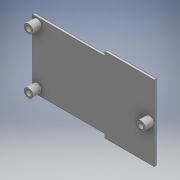
# Autodesk Inventor part: TopChassis
Saved by Autodesk Inventor 2016 (Build 200138000, 138)
## iProperties
Created: 2016-02-18
Part Number: TopChassis
Material: Generic
Document SubType Name: Modeling
Designer: mkepler
Density: 1 g/cm^3
Appearance: Default
Author: mkepler
Autodesk Inventor part; units mm, degrees
ref_plane "YZ Plane" through (0, 0, 0) normal (1, 0, 0) x (0, 1, 0)
ref_plane "XZ Plane" through (0, 0, 0) normal (0, 1, 0) x (-1, 0, 0)
ref_plane "XY Plane" through (0, 0, 0) normal (0, 0, 1) x (1, 0, 0)
sketch "Sketch1" plane through (0, 0, 0) normal (0, 1, 0) x (-1, 0, 0)
  line L0 (0, 0) -> (56, 0)
  line L1 (137.742, -4.5) -> (137.742, -80.5)
  line L2 (56, -85) -> (0, -85)
  line L3 (0, -85) -> (0, 0)
  line L4 (0, 0) -> (56, 0)
  line L5 (56, 0) -> (56, -4.5)
  line L6 (56, -85) -> (56, -80.5)
  line L7 (56, -80.5) -> (137.742, -80.5)
  line L8 (56, -4.5) -> (137.742, -4.5)
  line L9 (56, 0) -> (56, -4.5)
  line L10 (56, -80.5) -> (56, -85)
  dimension "d19" = 56
  dimension "d20" = 4.5
  dimension "d21" = 4.5
  dimension "d54" = 76
  dimension "d55" = 81.742
  dimension "d56" = 85
  constraints: 22 end point, 6 perpendicular, 1 horizontal, 1 vertical
  measures "d19" distance of L0.end L0.start
  measures "d20" distance of L0.end L5.end
  measures "d21" distance of L2.start L6.end
  measures "d54" distance between parallel lines of L7 L8
  measures "d55" distance between parallel lines of L1 L6
  measures "d56" distance between parallel lines of L2 L0
extrude "Extrusion1" add sketch "Sketch1" along normal blind 2.5
sketch "Sketch3" plane through (0, 2.5, 0) normal (0, 1, 0) x (1, 0, 0)
  line L0 (-56, 85) -> (-56, 80.5) projected
  line L1 (0, 0) -> (0, 85) projected
  circle A0 centre (-131.742, 10.5) radius 2.2
  line L2 (-137.742, 80.5) -> (-137.742, 4.5) projected
  line L3 (-137.742, 4.5) -> (-56, 4.5) projected
  line L4 (-131.742, 10.5) -> (-72.242, 10.5)
  line L5 (-101.992, 10.5) -> (-101.992, 4.5)
  circle A1 centre (-72.242, 10.5) radius 2.2
  line L6 (-72.242, 10.5) -> (-72.242, 28.5)
  circle A2 centre (-72.242, 28.5) radius 2.2
  circle A3 centre (-131.742, 28.5) radius 2.2
  point P0 (-56, 88)
  dimension "d22" = 56
  dimension "d23" = 4.4
  dimension "d24" = 6
  dimension "d25" = 6
  dimension "d26" = 59.5
  dimension "d28" = 18
  dimension "d29" = 4.4
  dimension "d42" = 4.4
  dimension "d43" = 4.4
  constraints: 6 end point, 4 centre point, 3 coincident, 2 symmetric about line, 1 horizontal, 1 midpoint, 1 perpendicular, 1 point on line, 1 vertical, 1 other
  measures "d22" distance between parallel lines of L0 L1
  measures "d23" diameter of A0
  measures "d24" distance from line of L2 L4.start
  measures "d25" distance from line of L3 L4.start
  measures "d26" distance of L4.start L4.end
  measures "d28" distance of L6.start L6.end
  measures "d29" diameter of A2
  measures "d42" diameter of A3
  measures "d43" diameter of A1
sketch "Sketch4" plane through (0, 0, 0) normal (0, -1, 0) x (1, 0, 0)
  line L0 (0, 0) -> (0, -85) projected
  line L1 (0, -42.5) -> (-5.074, -42.5)
  circle A0 centre (-5.074, -42.5) radius 3
  circle A1 centre (-5.074, -42.5) radius 5
  circle A2 centre (-132.242, -74) radius 3
  line L2 (-56, -80.5) -> (-137.742, -80.5) projected
  line L3 (-137.742, -80.5) -> (-137.742, -4.5) projected
  circle A3 centre (-132.242, -74) radius 5
  circle A4 centre (-132.242, -11) radius 3
  circle A5 centre (-132.242, -11) radius 5
  line L4 (-137.742, -4.5) -> (-56, -4.5) projected
  dimension "d33" = 5.074
  dimension "d34" = 6
  dimension "d35" = 10
  dimension "d36" = 6
  dimension "d37" = 6.5
  dimension "d38" = 5.5
  dimension "d39" = 10
  dimension "d57" = 63
  dimension "d58" = 6.5
  dimension "d59" = 5.5
  constraints: 6 centre point, 4 coincident, 2 end point, 1 horizontal, 1 midpoint
  measures "d33" distance of L1.start L1.end
  measures "d34" diameter of A0
  measures "d35" diameter of A1
  measures "d36" diameter of A2
  measures "d37" distance from line of A2.centre L2
  measures "d38" distance from line of L3 A2.centre
  measures "d39" diameter of A3
  measures "d57" distance of A2.centre A5.centre
  measures "d58" distance from line of L4 A5.centre
  measures "d59" distance from line of L3 A5.centre
extrude "Extrusion3" add sketch "Sketch4" along normal blind 10
hole "Hole1" at (-72.242, 2.5, -28.5) at (-72.242, 2.5, -10.5) at (-131.742, 2.5, -10.5) at (-131.742, 2.5, -28.5) direction (0, -1, 0) diameter 4.5 depth 2
body "Solid1"
